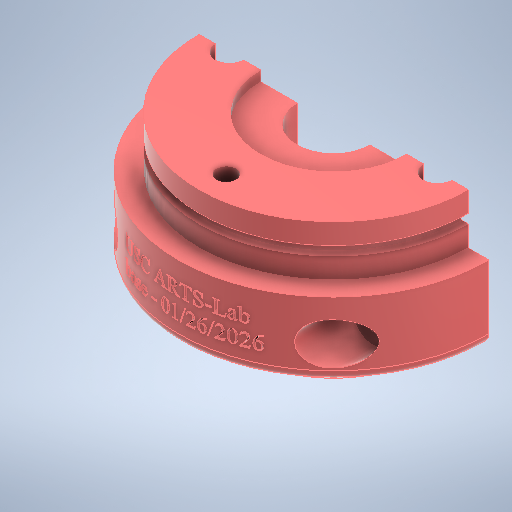
# Autodesk Inventor part: base_v0.7.0
Saved by Autodesk Inventor 2025 (Build 290162000, 162)
## iProperties
Created: 2026-01-12
Part Number: base_v0.7.0
Material: ABS Plastic
Document SubType Name: Modeling
Designer: SLM30
Density: 1.06 g/cm^3
Appearance: Smooth - Red
Author: SLM30
Autodesk Inventor part; units mm, degrees
ref_plane "YZ Plane" through (0, 0, 0) normal (1, 0, 0) x (0, 1, 0)
ref_plane "XZ Plane" through (0, 0, 0) normal (0, 1, 0) x (-1, 0, 0)
sketch "Sketch1" plane through (0, 0, 0) normal (0, 0, 1) x (1, 0, 0)
  line L0 (0, 0) -> (-14, 0)
  line L1 (-14, 0) -> (-14, 2)
  line L2 (-14, 2) -> (-25.825, 2)
  line L3 (-25.825, 2) -> (-25.825, -7.7)
  line L4 (-25.825, -7.7) -> (-29.825, -7.7)
  line L5 (0, 0) -> (0, -15)
  line L6 (0, -15) -> (-16, -15)
  line L7 (-16, -15) -> (-16, -26)
  line L8 (-16, -26) -> (0, -26)
  line L9 (0, -26) -> (0, -31)
  line L10 (0, -31) -> (-16, -31)
  line L11 (-29.825, -7.7) -> (-29.825, -21)
  line L12 (-29.825, -21) -> (-16, -31)
  arc A0 (-24.6268, -3.7009) -> (-24.6268, -2.0009) centre (-25.325, -2.8509) ccw
  line L13 (-25.825, -2.0009) -> (-24.6268, -2.0009)
  line L14 (-25.825, -3.7009) -> (-24.6268, -3.7009)
  line L15 (0, -37.6) -> (0, 8.6) projected
  dimension "d0" = 14
  dimension "d1" = 2
  dimension "d2" = 11.825
  dimension "d3" = 9.7
  dimension "d4" = 4
  dimension "d5" = 15
  dimension "d6" = 16
  dimension "d7" = 11
  dimension "d8" = 5
  dimension "d9" = 13.825
  dimension "d10" = 125.879
  dimension "d11" = 1.7
  dimension "d12" = 1.1
  dimension "d13" = 0.5
  dimension "d14" = 0.85
  dimension "d15" = 4.0009
  constraints: 30 end point, 7 perpendicular, 4 point on line, 3 horizontal, 2 point on circle, 2 vertical, 1 centre point, 1 parallel
  measures "d0" distance of L0.start L0.end
  measures "d1" distance of L0.end L1.end
  measures "d2" distance of L1.end L2.end
  measures "d3" distance of L2.end L3.end
  measures "d4" distance of L3.end L4.end
  measures "d5" distance of L0.start L5.end
  measures "d6" distance of L5.end L6.end
  measures "d7" distance of L6.end L7.end
  measures "d8" distance of L8.end L9.end
  measures "d9" horizontal distance of L11.end L10.end
  measures "d10" angle of L11 L12
  measures "d11" distance of L14.start L13.start
  measures "d12" radius of A0
  measures "d13" distance from line of L3 A0.centre
  measures "d14" distance from line of L14 A0.centre
  measures "d15" distance between parallel lines of L2 L13
revolve "Revolution1" add sketch "Sketch1" angle 180 about axis through (0, -10, 0) along (0, 1, 0) contours L5 L6 L7 L8 L9 L10 L12 L11 L4 L3 L14 A0 L13 L2 L1 L0
sketch "Sketch2" plane through (16, -31, 0) normal (0, 0, -1) x (-1, 0, 0)
  circle A0 centre (6, 10.5) radius 2.25
  line L0 (0, 5) -> (0, 16) projected
  line L1 (32, 16) -> (0, 16) projected
  point P0 (16, 31)
  dimension "d17" = 4.5
  dimension "d18" = 6
  dimension "d19" = 5.5
  constraints: 1 centre point
  measures "d17" diameter of A0
  measures "d18" distance from line of L0 A0.centre
  measures "d19" distance from line of L1 A0.centre
hole "Hole1" at (10, -20.5, 0) direction (0, 0, 1) diameter 4.5 depth 21.25
mirror "Mirror1" about plane through (0, 0, 0) normal (1, 0, 0) of "Hole1"
sketch "Sketch3" plane through (0, 0, 0) normal (0, 1, 0) x (1, 0, 0)
  circle A0 centre (0, 0) radius 7
  dimension "d27" = 14
  constraints: 1 centre point, 1 coincident
  measures "d27" diameter of A0
hole "Hole2" at (0, 0, 0) direction (0, -1, 0) diameter 14 depth 15
sketch "Sketch4" plane through (-16, -31, 0) normal (0, -1, 0) x (1, 0, 0)
  circle A0 centre (16, 0) radius 7
  point P0 (16, 0)
  dimension "d35" = 14
  constraints: 1 centre point, 1 coincident
  measures "d35" diameter of A0
hole "Hole3" at (0, -31, 0) direction (0, 1, 0) diameter 14 depth 10
ref_plane "Work Plane1" through (0, 0, 30) normal (0, 0, 1) x (1, 0, 0)
sketch "Sketch8" plane through (25.825, 2, 0) normal (0, 0, -1) x (-1, 0, 0)
  circle A0 centre (4.825, -17.5) radius 1.75
  line L0 (55.65, -23) -> (-4, -23) projected
  line L1 (9.825, -28) -> (9.825, -17) projected
  point P0 (25.825, -2)
  point P1 (-4, -23)
  dimension "d78" = 3.5
  dimension "d79" = 5.5
  dimension "d80" = 5
  constraints: 1 centre point, 1 other
  measures "d78" diameter of A0
  measures "d80" distance from line of L1 A0.centre
hole "Hole7" at (21, -15.5, 0) direction (0, 0, 1) diameter 3.5 end through all
mirror "Mirror2" about plane through (0, 0, 0) normal (1, 0, 0) of "Hole7"
sketch "Sketch9" plane through (0, 0, 30) normal (0, 0, 1) x (1, 0, 0)
  circle A0 centre (-21, -15.5) radius 1.75 projected
  circle A1 centre (-21, -15.5) radius 4
  point P0 (0, 0)
  dimension "d88" = 8
  constraints: 1 centre point, 1 coincident
  measures "d88" diameter of A1
hole "Hole8" at (-21, -15.5, 30) direction (0, 0, -1) diameter 8 depth 14
mirror "Mirror3" about plane through (0, 0, 0) normal (1, 0, 0) of "Hole8"
sketch "Sketch10" plane through (0, 0, 30) normal (0, 0, 1) x (1, 0, 0)
  circle A0 centre (-21, -15.5) radius 1.75 projected
  line L0 (-18.8265, -17.7354) -> (-21.8492, -18.5)
  line L1 (-21.8492, -18.5) -> (-24.0227, -16.2646)
  line L2 (-24.0227, -16.2646) -> (-23.1735, -13.2646)
  line L3 (-23.1735, -13.2646) -> (-20.1508, -12.5)
  line L4 (-20.1508, -12.5) -> (-17.9773, -14.7354)
  line L5 (-17.9773, -14.7354) -> (-18.8265, -17.7354)
  point P0 (0, 0)
  dimension "d135" = 3
  constraints: 12 end point, 1 coincident, 13 other
  measures "d135" vertical distance of L4.end L0.start
extrude "Extrusion1" cut sketch "Sketch10" against normal blind 16
fillet "Fillet1" radius 2 1 edges at (0, -21, 29.825)
sketch "Sketch16" plane through (-25.825, 2, 0) normal (0, 1, 0) x (1, 0, 0)
  circle A0 centre (25.825, -20.615) radius 1.9085
  arc A1 (0, 0) -> (51.65, 0) centre (25.825, 0) ccw projected
  point P0 (25.825, 0)
  point P1 (25.825, -25.825)
  dimension "d108" = 3.817
  dimension "d109" = 20.615
  dimension "d110" = 5.21
  constraints: 1 centre point, 1 point on circle
  measures "d108" diameter of A0
  measures "d109" distance of point (25.825, 0) A0.centre
  measures "d110" distance of point (25.825, -25.825) A0.centre
hole "Hole9" at (0, 2, 20.615) direction (0, -1, 0) diameter 3.817 end through all
sketch "Sketch17" plane through (-16, -31, 0) normal (0, -1, 0) x (1, 0, 0)
  circle A0 centre (16, 20.615) radius 1.9085 projected
  circle A1 centre (16, 20.615) radius 3
  point P0 (16, 0)
  dimension "d118" = 6
  constraints: 1 centre point, 1 coincident
  measures "d118" diameter of A1
hole "Hole10" at (0, -31, 20.615) direction (0, 1, 0) diameter 6 depth 7
sketch "Sketch18" plane through (-25.825, 2, 0) normal (0, 1, 0) x (1, 0, 0)
  circle A0 centre (5.825, 0) radius 2.75
  point P0 (25.825, 0)
  dimension "d126" = 5.5
  dimension "d127" = 20
  constraints: 1 centre point
  measures "d126" diameter of A0
  measures "d127" distance of point (25.825, 0) A0.centre
hole "Hole11" at (-20, 2, 0) direction (0, -1, 0) diameter 5.5 depth 3.3
mirror "Mirror5" about plane through (0, 0, 0) normal (1, 0, 0) of "Hole11"
move faces "Move1" translate (0, 0, -2.5) faces at (20.5413, -18.6943, 16) (17.0002, -15.4615, 18.8349)
ref_plane "Work Plane3" through (0, -14.35, 29.825) normal (0, 0, 1) x (1, 0, 0)
sketch "Sketch19" plane through (0, -14.35, 29.825) normal (0, 0, 1) x (1, 0, 0)
  line L0 (-29.825, 6.65) -> (-29.825, -5.6283) projected
  line L1 (-11.7404, 3.0074) -> (-11.7404, 3.0759)
  line L2 (-11.7404, 3.0759) -> (-10.846, 3.0759)
  line L3 (-10.846, 3.0759) -> (-10.846, 3.0074)
  line L4 (-10.846, 3.0074) -> (-10.9415, 3.0074)
  spline S0 degree 2 poles (-10.9415, 3.0074) (-11.0909, 3.0074) (-11.1697, 2.8808) knots 0 0 0 1 1 1
  spline S1 degree 2 poles (-11.1697, 2.8808) (-11.2092, 2.8227) (-11.2092, 2.611) knots 0 0 0 1 1 1
  line L5 (-11.2092, 2.611) -> (-11.2092, 1.5818)
  spline S2 degree 2 poles (-11.2092, 1.5818) (-11.2092, 1.1999) (-11.3606, 0.7787) (-11.8047, 0.4778) (-12.1866, 0.4778) knots 0 0 0 1 2 3 3 3
  spline S3 degree 2 poles (-12.1866, 0.4778) (-12.6016, 0.4778) (-13.0332, 0.7662) (-13.1225, 1.009) knots 0 0 0 1 2 2 2
  spline S4 degree 2 poles (-13.1225, 1.009) (-13.1826, 1.175) (-13.1826, 1.6336) knots 0 0 0 1 1 1
  line L6 (-13.1826, 1.6336) -> (-13.1826, 2.6256)
  spline S5 degree 2 poles (-13.1826, 2.6256) (-13.1826, 2.8601) (-13.3113, 3.0074) (-13.4566, 3.0074) knots 0 0 0 1 2 2 2
  line L7 (-13.4566, 3.0074) -> (-13.552, 3.0074)
  line L8 (-13.552, 3.0074) -> (-13.552, 3.0759)
  line L9 (-13.552, 3.0759) -> (-12.4543, 3.0759)
  line L10 (-12.4543, 3.0759) -> (-12.4543, 3.0074)
  line L11 (-12.4543, 3.0074) -> (-12.5518, 3.0074)
  spline S6 degree 2 poles (-12.5518, 3.0074) (-12.7095, 3.0074) (-12.7759, 2.9078) knots 0 0 0 1 1 1
  spline S7 degree 2 poles (-12.7759, 2.9078) (-12.8236, 2.8393) (-12.8236, 2.6256) knots 0 0 0 1 1 1
  line L12 (-12.8236, 2.6256) -> (-12.8236, 1.5195)
  spline S8 degree 2 poles (-12.8236, 1.5195) (-12.8236, 1.3722) (-12.7697, 0.9903) (-12.6265, 0.7787) (-12.3588, 0.6396) (-12.1637, 0.6396) knots 0 0 0 1 2 3 4 4 4
  spline S9 degree 2 poles (-12.1637, 0.6396) (-11.9147, 0.6396) (-11.5225, 0.8575) (-11.3772, 1.1958) (-11.3772, 1.5984) knots 0 0 0 1 2 3 3 3
  line L13 (-11.3772, 1.5984) -> (-11.3772, 2.6256)
  spline S10 degree 2 poles (-11.3772, 2.6256) (-11.3772, 2.8642) (-11.4291, 2.9244) knots 0 0 0 1 1 1
  spline S11 degree 2 poles (-11.4291, 2.9244) (-11.5018, 3.0074) (-11.6449, 3.0074) knots 0 0 0 1 1 1
  line L14 (-11.6449, 3.0074) -> (-11.7404, 3.0074)
  line L15 (-9.0385, 3.134) -> (-9.0385, 2.2562)
  line L16 (-9.0385, 2.2562) -> (-9.107, 2.2562)
  spline S12 degree 2 poles (-9.107, 2.2562) (-9.1402, 2.5094) (-9.3166, 2.8082) (-9.6383, 2.9846) (-9.8126, 2.9846) knots 0 0 0 1 2 3 3 3
  spline S13 degree 2 poles (-9.8126, 2.9846) (-10.0076, 2.9846) (-10.2629, 2.7459) (-10.2629, 2.5944) knots 0 0 0 1 2 2 2
  spline S14 degree 2 poles (-10.2629, 2.5944) (-10.2629, 2.4782) (-10.1819, 2.3828) knots 0 0 0 1 1 1
  spline S15 degree 2 poles (-10.1819, 2.3828) (-10.0657, 2.2417) (-9.6279, 2.0072) knots 0 0 0 1 1 1
  spline S16 degree 2 poles (-9.6279, 2.0072) (-9.273, 1.8163) (-9.0116, 1.6129) (-8.8704, 1.3348) (-8.8704, 1.1833) knots 0 0 0 1 2 3 3 3
  spline S17 degree 2 poles (-8.8704, 1.1833) (-8.8704, 0.8949) (-9.3187, 0.4778) (-9.6715, 0.4778) knots 0 0 0 1 2 2 2
  spline S18 degree 2 poles (-9.6715, 0.4778) (-9.7814, 0.4778) (-9.879, 0.4944) knots 0 0 0 1 1 1
  spline S19 degree 2 poles (-9.879, 0.4944) (-9.9371, 0.5048) (-10.3023, 0.623) (-10.3521, 0.623) knots 0 0 0 1 2 2 2
  spline S20 degree 2 poles (-10.3521, 0.623) (-10.3978, 0.623) (-10.4538, 0.567) (-10.4662, 0.4778) knots 0 0 0 1 2 2 2
  line L17 (-10.4662, 0.4778) -> (-10.5347, 0.4778)
  line L18 (-10.5347, 0.4778) -> (-10.5347, 1.3493)
  line L19 (-10.5347, 1.3493) -> (-10.4662, 1.3493)
  spline S21 degree 2 poles (-10.4662, 1.3493) (-10.4185, 1.0754) (-10.2525, 0.8036) (-9.9122, 0.623) (-9.7109, 0.623) knots 0 0 0 1 2 3 3 3
  spline S22 degree 2 poles (-9.7109, 0.623) (-9.4764, 0.623) (-9.2045, 0.87) (-9.2045, 1.0401) knots 0 0 0 1 2 2 2
  spline S23 degree 2 poles (-9.2045, 1.0401) (-9.2045, 1.1335) (-9.3083, 1.3244) (-9.4162, 1.4075) knots 0 0 0 1 2 2 2
  spline S24 degree 2 poles (-9.4162, 1.4075) (-9.4888, 1.4635) (-10.1425, 1.8287) (-10.4185, 2.0466) (-10.5617, 2.3081) (-10.5617, 2.4658) knots 0 0 0 1 2 3 4 4 4
  spline S25 degree 2 poles (-10.5617, 2.4658) (-10.5617, 2.7397) (-10.1404, 3.134) (-9.8146, 3.134) knots 0 0 0 1 2 2 2
  spline S26 degree 2 poles (-9.8146, 3.134) (-9.6134, 3.134) (-9.3851, 3.0344) knots 0 0 0 1 1 1
  spline S27 degree 2 poles (-9.3851, 3.0344) (-9.2793, 2.9887) (-9.2357, 2.9887) knots 0 0 0 1 1 1
  spline S28 degree 2 poles (-9.2357, 2.9887) (-9.1879, 2.9887) (-9.1257, 3.0468) (-9.107, 3.134) knots 0 0 0 1 2 2 2
  line L20 (-9.107, 3.134) -> (-9.0385, 3.134)
  line L21 (-6.3595, 3.134) -> (-6.3014, 2.2707)
  line L22 (-6.3014, 2.2707) -> (-6.3595, 2.2707)
  spline S29 degree 2 poles (-6.3595, 2.2707) (-6.4757, 2.6588) (-6.9053, 3.0012) (-7.2062, 3.0012) knots 0 0 0 1 2 2 2
  spline S30 degree 2 poles (-7.2062, 3.0012) (-7.4573, 3.0012) (-7.864, 2.7439) (-8.0985, 2.1815) (-8.0985, 1.7623) knots 0 0 0 1 2 3 3 3
  spline S31 degree 2 poles (-8.0985, 1.7623) (-8.0985, 1.4178) (-7.8785, 0.9115) (-7.4344, 0.6417) (-7.1522, 0.6417) knots 0 0 0 1 2 3 3 3
  spline S32 degree 2 poles (-7.1522, 0.6417) (-6.9053, 0.6417) (-6.5276, 0.8534) (-6.3014, 1.1688) knots 0 0 0 1 2 2 2
  line L23 (-6.3014, 1.1688) -> (-6.2433, 1.1315)
  spline S33 degree 2 poles (-6.2433, 1.1315) (-6.4342, 0.7932) (-6.9426, 0.4778) (-7.2933, 0.4778) knots 0 0 0 1 2 2 2
  spline S34 degree 2 poles (-7.2933, 0.4778) (-7.9242, 0.4778) (-8.2707, 0.9468) knots 0 0 0 1 1 1
  spline S35 degree 2 poles (-8.2707, 0.9468) (-8.528, 1.2954) (-8.528, 1.7665) knots 0 0 0 1 1 1
  spline S36 degree 2 poles (-8.528, 1.7665) (-8.528, 2.1462) (-8.1877, 2.7833) (-7.5901, 3.134) (-7.2373, 3.134) knots 0 0 0 1 2 3 3 3
  spline S37 degree 2 poles (-7.2373, 3.134) (-6.9634, 3.134) (-6.6957, 2.9991) knots 0 0 0 1 1 1
  spline S38 degree 2 poles (-6.6957, 2.9991) (-6.6168, 2.9576) (-6.5836, 2.9576) knots 0 0 0 1 1 1
  spline S39 degree 2 poles (-6.5836, 2.9576) (-6.5317, 2.9576) (-6.4944, 2.9929) knots 0 0 0 1 1 1
  spline S40 degree 2 poles (-6.4944, 2.9929) (-6.4467, 3.0448) (-6.4259, 3.134) knots 0 0 0 1 1 1
  line L24 (-6.4259, 3.134) -> (-6.3595, 3.134)
  line L25 (-3.392, 1.3846) -> (-4.3798, 1.3846)
  line L26 (-4.3798, 1.3846) -> (-4.552, 0.9862)
  spline S41 degree 2 poles (-4.552, 0.9862) (-4.6164, 0.8368) (-4.6164, 0.7641) knots 0 0 0 1 1 1
  spline S42 degree 2 poles (-4.6164, 0.7641) (-4.6164, 0.706) (-4.5043, 0.6168) (-4.3217, 0.6044) knots 0 0 0 1 2 2 2
  line L27 (-4.3217, 0.6044) -> (-4.3217, 0.5359)
  line L28 (-4.3217, 0.5359) -> (-5.1227, 0.5359)
  line L29 (-5.1227, 0.5359) -> (-5.1227, 0.6044)
  spline S43 degree 2 poles (-5.1227, 0.6044) (-4.9629, 0.6334) (-4.9173, 0.677) knots 0 0 0 1 1 1
  spline S44 degree 2 poles (-4.9173, 0.677) (-4.8218, 0.7683) (-4.7056, 1.0443) knots 0 0 0 1 1 1
  line L30 (-4.7056, 1.0443) -> (-3.8091, 3.134)
  line L31 (-3.8091, 3.134) -> (-3.7427, 3.134)
  line L32 (-3.7427, 3.134) -> (-2.8587, 1.0215)
  spline S45 degree 2 poles (-2.8587, 1.0215) (-2.7529, 0.7662) (-2.5786, 0.6147) (-2.4229, 0.6044) knots 0 0 0 1 2 2 2
  line L33 (-2.4229, 0.6044) -> (-2.4229, 0.5359)
  line L34 (-2.4229, 0.5359) -> (-3.4252, 0.5359)
  line L35 (-3.4252, 0.5359) -> (-3.4252, 0.6044)
  spline S46 degree 2 poles (-3.4252, 0.6044) (-3.2737, 0.6127) (-3.1658, 0.6977) (-3.1658, 0.76) knots 0 0 0 1 2 2 2
  spline S47 degree 2 poles (-3.1658, 0.76) (-3.1658, 0.843) (-3.2405, 1.0215) knots 0 0 0 1 1 1
  line L36 (-3.2405, 1.0215) -> (-3.392, 1.3846)
  line L37 (-3.4501, 1.5237) -> (-3.8776, 2.5509)
  line L38 (-3.8776, 2.5509) -> (-4.3217, 1.5237)
  line L39 (-4.3217, 1.5237) -> (-3.4501, 1.5237)
  line L40 (0.2125, 0.5359) -> (-0.466, 0.5359)
  line L41 (-0.466, 0.5359) -> (-1.3272, 1.7229)
  spline S48 degree 2 poles (-1.3272, 1.7229) (-1.4227, 1.7187) (-1.4808, 1.7187) knots 0 0 0 1 1 1
  spline S49 degree 2 poles (-1.4808, 1.7187) (-1.5057, 1.7187) (-1.5617, 1.7208) (-1.5908, 1.7229) knots 0 0 0 1 2 2 2
  line L42 (-1.5908, 1.7229) -> (-1.5908, 0.9862)
  spline S50 degree 2 poles (-1.5908, 0.9862) (-1.5908, 0.7455) (-1.5389, 0.6874) knots 0 0 0 1 1 1
  spline S51 degree 2 poles (-1.5389, 0.6874) (-1.4683, 0.6044) (-1.3272, 0.6044) knots 0 0 0 1 1 1
  line L43 (-1.3272, 0.6044) -> (-1.2276, 0.6044)
  line L44 (-1.2276, 0.6044) -> (-1.2276, 0.5359)
  line L45 (-1.2276, 0.5359) -> (-2.3129, 0.5359)
  line L46 (-2.3129, 0.5359) -> (-2.3129, 0.6044)
  line L47 (-2.3129, 0.6044) -> (-2.2175, 0.6044)
  spline S52 degree 2 poles (-2.2175, 0.6044) (-2.0577, 0.6044) (-1.9892, 0.7102) knots 0 0 0 1 1 1
  spline S53 degree 2 poles (-1.9892, 0.7102) (-1.9498, 0.7683) (-1.9498, 0.9862) knots 0 0 0 1 1 1
  line L48 (-1.9498, 0.9862) -> (-1.9498, 2.6256)
  spline S54 degree 2 poles (-1.9498, 2.6256) (-1.9498, 2.8663) (-2.0017, 2.9244) knots 0 0 0 1 1 1
  spline S55 degree 2 poles (-2.0017, 2.9244) (-2.0743, 3.0074) (-2.2175, 3.0074) knots 0 0 0 1 1 1
  line L49 (-2.2175, 3.0074) -> (-2.3129, 3.0074)
  line L50 (-2.3129, 3.0074) -> (-2.3129, 3.0759)
  line L51 (-2.3129, 3.0759) -> (-1.3895, 3.0759)
  spline S56 degree 2 poles (-1.3895, 3.0759) (-0.9848, 3.0759) (-0.6009, 2.9576) (-0.3332, 2.6422) (-0.3332, 2.4222) knots 0 0 0 1 2 3 3 3
  spline S57 degree 2 poles (-0.3332, 2.4222) (-0.3332, 2.1877) (-0.6383, 1.8432) (-0.9599, 1.7727) knots 0 0 0 1 2 2 2
  line L52 (-0.9599, 1.7727) -> (-0.4328, 1.0443)
  spline S58 degree 2 poles (-0.4328, 1.0443) (-0.2523, 0.7932) (0.005, 0.6272) (0.2125, 0.6044) knots 0 0 0 1 2 2 2
  line L53 (0.2125, 0.6044) -> (0.2125, 0.5359)
  spline S59 degree 2 poles (-1.5908, 1.8412) (-1.5555, 1.8412) (-1.5036, 1.8391) (-1.487, 1.8391) knots 0 0 0 1 2 2 2
  spline S60 degree 2 poles (-1.487, 1.8391) (-1.128, 1.8391) (-0.7628, 2.1545) (-0.7628, 2.3973) knots 0 0 0 1 2 2 2
  spline S61 degree 2 poles (-0.7628, 2.3973) (-0.7628, 2.6359) (-1.0575, 2.9327) (-1.3003, 2.9327) knots 0 0 0 1 2 2 2
  spline S62 degree 2 poles (-1.3003, 2.9327) (-1.4082, 2.9327) (-1.5908, 2.8974) knots 0 0 0 1 1 1
  line L54 (-1.5908, 2.8974) -> (-1.5908, 1.8412)
  line L55 (2.3956, 3.0759) -> (2.4226, 2.4803)
  line L56 (2.4226, 2.4803) -> (2.352, 2.4803)
  spline S63 degree 2 poles (2.352, 2.4803) (2.3313, 2.6359) (2.296, 2.7044) knots 0 0 0 1 1 1
  spline S64 degree 2 poles (2.296, 2.7044) (2.2379, 2.8123) (2.0449, 2.9161) (1.8872, 2.9161) knots 0 0 0 1 2 2 2
  line L57 (1.8872, 2.9161) -> (1.5303, 2.9161)
  line L58 (1.5303, 2.9161) -> (1.5303, 0.9758)
  spline S65 degree 2 poles (1.5303, 0.9758) (1.5303, 0.7413) (1.5801, 0.6832) knots 0 0 0 1 1 1
  spline S66 degree 2 poles (1.5801, 0.6832) (1.6527, 0.6044) (1.8, 0.6044) knots 0 0 0 1 1 1
  line L59 (1.8, 0.6044) -> (1.8872, 0.6044)
  line L60 (1.8872, 0.6044) -> (1.8872, 0.5359)
  line L61 (1.8872, 0.5359) -> (0.8123, 0.5359)
  line L62 (0.8123, 0.5359) -> (0.8123, 0.6044)
  line L63 (0.8123, 0.6044) -> (0.9015, 0.6044)
  spline S67 degree 2 poles (0.9015, 0.6044) (1.0634, 0.6044) (1.1298, 0.7019) knots 0 0 0 1 1 1
  spline S68 degree 2 poles (1.1298, 0.7019) (1.1713, 0.7621) (1.1713, 0.9758) knots 0 0 0 1 1 1
  line L64 (1.1713, 0.9758) -> (1.1713, 2.9161)
  line L65 (1.1713, 2.9161) -> (0.8662, 2.9161)
  spline S69 degree 2 poles (0.8662, 2.9161) (0.6878, 2.9161) (0.6131, 2.8891) knots 0 0 0 1 1 1
  spline S70 degree 2 poles (0.6131, 2.8891) (0.5155, 2.8538) (0.3786, 2.6525) (0.364, 2.4803) knots 0 0 0 1 2 2 2
  line L66 (0.364, 2.4803) -> (0.2935, 2.4803)
  line L67 (0.2935, 2.4803) -> (0.3225, 3.0759)
  line L68 (0.3225, 3.0759) -> (2.3956, 3.0759)
  line L69 (4.284, 3.134) -> (4.284, 2.2562)
  line L70 (4.284, 2.2562) -> (4.2155, 2.2562)
  spline S71 degree 2 poles (4.2155, 2.2562) (4.1823, 2.5094) (4.0059, 2.8082) (3.6843, 2.9846) (3.51, 2.9846) knots 0 0 0 1 2 3 3 3
  spline S72 degree 2 poles (3.51, 2.9846) (3.3149, 2.9846) (3.0597, 2.7459) (3.0597, 2.5944) knots 0 0 0 1 2 2 2
  spline S73 degree 2 poles (3.0597, 2.5944) (3.0597, 2.4782) (3.1406, 2.3828) knots 0 0 0 1 1 1
  spline S74 degree 2 poles (3.1406, 2.3828) (3.2568, 2.2417) (3.6947, 2.0072) knots 0 0 0 1 1 1
  spline S75 degree 2 poles (3.6947, 2.0072) (4.0495, 1.8163) (4.311, 1.6129) (4.4521, 1.3348) (4.4521, 1.1833) knots 0 0 0 1 2 3 3 3
  spline S76 degree 2 poles (4.4521, 1.1833) (4.4521, 0.8949) (4.0039, 0.4778) (3.6511, 0.4778) knots 0 0 0 1 2 2 2
  spline S77 degree 2 poles (3.6511, 0.4778) (3.5411, 0.4778) (3.4436, 0.4944) knots 0 0 0 1 1 1
  spline S78 degree 2 poles (3.4436, 0.4944) (3.3855, 0.5048) (3.0202, 0.623) (2.9704, 0.623) knots 0 0 0 1 2 2 2
  spline S79 degree 2 poles (2.9704, 0.623) (2.9248, 0.623) (2.8688, 0.567) (2.8563, 0.4778) knots 0 0 0 1 2 2 2
  line L71 (2.8563, 0.4778) -> (2.7878, 0.4778)
  line L72 (2.7878, 0.4778) -> (2.7878, 1.3493)
  line L73 (2.7878, 1.3493) -> (2.8563, 1.3493)
  spline S80 degree 2 poles (2.8563, 1.3493) (2.904, 1.0754) (3.07, 0.8036) (3.4104, 0.623) (3.6117, 0.623) knots 0 0 0 1 2 3 3 3
  spline S81 degree 2 poles (3.6117, 0.623) (3.8462, 0.623) (4.118, 0.87) (4.118, 1.0401) knots 0 0 0 1 2 2 2
  spline S82 degree 2 poles (4.118, 1.0401) (4.118, 1.1335) (4.0142, 1.3244) (3.9063, 1.4075) knots 0 0 0 1 2 2 2
  spline S83 degree 2 poles (3.9063, 1.4075) (3.8337, 1.4635) (3.18, 1.8287) (2.904, 2.0466) (2.7608, 2.3081) (2.7608, 2.4658) knots 0 0 0 1 2 3 4 4 4
  spline S84 degree 2 poles (2.7608, 2.4658) (2.7608, 2.7397) (3.1821, 3.134) (3.5079, 3.134) knots 0 0 0 1 2 2 2
  spline S85 degree 2 poles (3.5079, 3.134) (3.7092, 3.134) (3.9375, 3.0344) knots 0 0 0 1 1 1
  spline S86 degree 2 poles (3.9375, 3.0344) (4.0433, 2.9887) (4.0869, 2.9887) knots 0 0 0 1 1 1
  spline S87 degree 2 poles (4.0869, 2.9887) (4.1346, 2.9887) (4.1969, 3.0468) (4.2155, 3.134) knots 0 0 0 1 2 2 2
  line L74 (4.2155, 3.134) -> (4.284, 3.134)
  line L75 (4.809, 1.5382) -> (5.7802, 1.5382)
  line L76 (5.7802, 1.5382) -> (5.7802, 1.256)
  line L77 (5.7802, 1.256) -> (4.809, 1.256)
  line L78 (4.809, 1.256) -> (4.809, 1.5382)
  line L79 (8.1314, 1.2394) -> (8.1936, 1.2269)
  line L80 (8.1936, 1.2269) -> (7.9757, 0.5359)
  line L81 (7.9757, 0.5359) -> (6.0106, 0.5359)
  line L82 (6.0106, 0.5359) -> (6.0106, 0.6044)
  line L83 (6.0106, 0.6044) -> (6.106, 0.6044)
  spline S88 degree 2 poles (6.106, 0.6044) (6.2658, 0.6044) (6.3343, 0.7102) knots 0 0 0 1 1 1
  spline S89 degree 2 poles (6.3343, 0.7102) (6.3737, 0.7683) (6.3737, 0.9862) knots 0 0 0 1 1 1
  line L84 (6.3737, 0.9862) -> (6.3737, 2.6256)
  spline S90 degree 2 poles (6.3737, 2.6256) (6.3737, 2.8642) (6.3218, 2.9244) knots 0 0 0 1 1 1
  spline S91 degree 2 poles (6.3218, 2.9244) (6.2492, 3.0074) (6.106, 3.0074) knots 0 0 0 1 1 1
  line L85 (6.106, 3.0074) -> (6.0106, 3.0074)
  line L86 (6.0106, 3.0074) -> (6.0106, 3.0759)
  line L87 (6.0106, 3.0759) -> (7.1581, 3.0759)
  line L88 (7.1581, 3.0759) -> (7.1581, 3.0074)
  spline S92 degree 2 poles (7.1581, 3.0074) (6.9548, 3.0095) (6.7929, 2.9306) (6.7327, 2.8103) (6.7327, 2.5841) knots 0 0 0 1 2 3 3 3
  line L89 (6.7327, 2.5841) -> (6.7327, 0.9883)
  spline S93 degree 2 poles (6.7327, 0.9883) (6.7327, 0.8326) (6.7618, 0.7745) knots 0 0 0 1 1 1
  spline S94 degree 2 poles (6.7618, 0.7745) (6.7846, 0.7351) (6.878, 0.6977) (7.1249, 0.6977) knots 0 0 0 1 2 2 2
  line L90 (7.1249, 0.6977) -> (7.3096, 0.6977)
  spline S95 degree 2 poles (7.3096, 0.6977) (7.6022, 0.6977) (7.8388, 0.7849) (8.0338, 1.0028) (8.1314, 1.2394) knots 0 0 0 1 2 3 3 3
  spline S96 degree 2 poles (9.3661, 0.7849) (9.1025, 0.5795) (9.0341, 0.5483) knots 0 0 0 1 1 1
  spline S97 degree 2 poles (9.0341, 0.5483) (8.9345, 0.5006) (8.8203, 0.5006) knots 0 0 0 1 1 1
  spline S98 degree 2 poles (8.8203, 0.5006) (8.6419, 0.5006) (8.4115, 0.7434) (8.4115, 0.9426) knots 0 0 0 1 2 2 2
  spline S99 degree 2 poles (8.4115, 0.9426) (8.4115, 1.0671) (8.4675, 1.1605) knots 0 0 0 1 1 1
  spline S100 degree 2 poles (8.4675, 1.1605) (8.5443, 1.2871) (8.9241, 1.5112) (9.3661, 1.6731) knots 0 0 0 1 2 2 2
  line L91 (9.3661, 1.6731) -> (9.3661, 1.7395)
  spline S101 degree 2 poles (9.3661, 1.7395) (9.3661, 1.9968) (9.2042, 2.1877) (9.0486, 2.1877) knots 0 0 0 1 2 2 2
  spline S102 degree 2 poles (9.0486, 2.1877) (8.9324, 2.1877) (8.8618, 2.1234) knots 0 0 0 1 1 1
  spline S103 degree 2 poles (8.8618, 2.1234) (8.7913, 2.0611) (8.7913, 1.9781) knots 0 0 0 1 1 1
  line L92 (8.7913, 1.9781) -> (8.7954, 1.8702)
  spline S104 degree 2 poles (8.7954, 1.8702) (8.7954, 1.7831) (8.7062, 1.6897) (8.6356, 1.6897) knots 0 0 0 1 2 2 2
  spline S105 degree 2 poles (8.6356, 1.6897) (8.5672, 1.6897) (8.4779, 1.7872) (8.4779, 1.8723) knots 0 0 0 1 2 2 2
  spline S106 degree 2 poles (8.4779, 1.8723) (8.4779, 2.0321) (8.8079, 2.3018) (9.1046, 2.3018) knots 0 0 0 1 2 2 2
  spline S107 degree 2 poles (9.1046, 2.3018) (9.3329, 2.3018) (9.4781, 2.2251) knots 0 0 0 1 1 1
  spline S108 degree 2 poles (9.4781, 2.2251) (9.5902, 2.167) (9.6421, 2.0445) knots 0 0 0 1 1 1
  spline S109 degree 2 poles (9.6421, 2.0445) (9.6753, 1.9636) (9.6753, 1.7146) knots 0 0 0 1 1 1
  line L93 (9.6753, 1.7146) -> (9.6753, 1.1315)
  spline S110 degree 2 poles (9.6753, 1.1315) (9.6753, 0.8866) (9.694, 0.7766) (9.7375, 0.7392) (9.7645, 0.7392) knots 0 0 0 1 2 3 3 3
  spline S111 degree 2 poles (9.7645, 0.7392) (9.7956, 0.7392) (9.8185, 0.7517) knots 0 0 0 1 1 1
  spline S112 degree 2 poles (9.8185, 0.7517) (9.8579, 0.7766) (9.97, 0.8887) knots 0 0 0 1 1 1
  line L94 (9.97, 0.8887) -> (9.97, 0.7849)
  spline S113 degree 2 poles (9.97, 0.7849) (9.7604, 0.5027) (9.5695, 0.5027) knots 0 0 0 1 1 1
  spline S114 degree 2 poles (9.5695, 0.5027) (9.4761, 0.5027) (9.3682, 0.6293) (9.3661, 0.7849) knots 0 0 0 1 2 2 2
  line L95 (9.3661, 0.9053) -> (9.3661, 1.5589)
  spline S115 degree 2 poles (9.3661, 1.5589) (9.0839, 1.4469) (9.0009, 1.3991) knots 0 0 0 1 1 1
  spline S116 degree 2 poles (9.0009, 1.3991) (8.8535, 1.3182) (8.7269, 1.1377) (8.7269, 1.0318) knots 0 0 0 1 2 2 2
  spline S117 degree 2 poles (8.7269, 1.0318) (8.7269, 0.897) (8.8867, 0.7185) (8.9926, 0.7185) knots 0 0 0 1 2 2 2
  spline S118 degree 2 poles (8.9926, 0.7185) (9.1337, 0.7185) (9.3661, 0.9053) knots 0 0 0 1 1 1
  spline S119 degree 2 poles (10.5697, 1.9532) (10.8187, 2.3018) (11.1051, 2.3018) knots 0 0 0 1 1 1
  spline S120 degree 2 poles (11.1051, 2.3018) (11.3686, 2.3018) (11.7608, 1.8515) (11.7608, 1.4593) knots 0 0 0 1 2 2 2
  spline S121 degree 2 poles (11.7608, 1.4593) (11.7608, 1.0028) (11.4579, 0.7226) knots 0 0 0 1 1 1
  spline S122 degree 2 poles (11.4579, 0.7226) (11.1985, 0.484) (10.8768, 0.484) knots 0 0 0 1 1 1
  spline S123 degree 2 poles (10.8768, 0.484) (10.7274, 0.484) (10.4203, 0.5919) (10.2584, 0.7019) knots 0 0 0 1 2 2 2
  line L96 (10.2584, 0.7019) -> (10.2584, 2.4782)
  spline S124 degree 2 poles (10.2584, 2.4782) (10.2584, 2.7688) (10.2294, 2.9036) (10.1713, 2.9514) (10.1256, 2.9514) knots 0 0 0 1 2 3 3 3
  spline S125 degree 2 poles (10.1256, 2.9514) (10.0737, 2.9514) (9.9949, 2.9223) knots 0 0 0 1 1 1
  line L97 (9.9949, 2.9223) -> (9.9679, 2.9908)
  line L98 (9.9679, 2.9908) -> (10.4846, 3.2004)
  line L99 (10.4846, 3.2004) -> (10.5697, 3.2004)
  line L100 (10.5697, 3.2004) -> (10.5697, 1.9532)
  line L101 (10.5697, 1.8349) -> (10.5697, 0.8098)
  spline S126 degree 2 poles (10.5697, 0.8098) (10.6651, 0.7164) (10.8685, 0.621) (10.9743, 0.621) knots 0 0 0 1 2 2 2
  spline S127 degree 2 poles (10.9743, 0.621) (11.1445, 0.621) (11.4371, 0.9945) (11.4371, 1.3514) knots 0 0 0 1 2 2 2
  spline S128 degree 2 poles (11.4371, 1.3514) (11.4371, 1.6814) (11.1445, 2.0341) (10.9577, 2.0341) knots 0 0 0 1 2 2 2
  spline S129 degree 2 poles (10.9577, 2.0341) (10.8581, 2.0341) (10.7606, 1.9843) knots 0 0 0 1 1 1
  spline S130 degree 2 poles (10.7606, 1.9843) (10.6859, 1.947) (10.5697, 1.8349) knots 0 0 0 1 1 1
  spline S131 degree 2 poles (-12.9813, -2.0642) (-12.7323, -1.7155) (-12.446, -1.7155) knots 0 0 0 1 1 1
  spline S132 degree 2 poles (-12.446, -1.7155) (-12.1824, -1.7155) (-11.7902, -2.1658) (-11.7902, -2.558) knots 0 0 0 1 2 2 2
  spline S133 degree 2 poles (-11.7902, -2.558) (-11.7902, -3.0146) (-12.0932, -3.2947) knots 0 0 0 1 1 1
  spline S134 degree 2 poles (-12.0932, -3.2947) (-12.3526, -3.5334) (-12.6742, -3.5334) knots 0 0 0 1 1 1
  spline S135 degree 2 poles (-12.6742, -3.5334) (-12.8236, -3.5334) (-13.1308, -3.4255) (-13.2926, -3.3155) knots 0 0 0 1 2 2 2
  line L102 (-13.2926, -3.3155) -> (-13.2926, -1.5391)
  spline S136 degree 2 poles (-13.2926, -1.5391) (-13.2926, -1.2486) (-13.3217, -1.1137) (-13.3798, -1.066) (-13.4254, -1.066) knots 0 0 0 1 2 3 3 3
  spline S137 degree 2 poles (-13.4254, -1.066) (-13.4773, -1.066) (-13.5562, -1.0951) knots 0 0 0 1 1 1
  line L103 (-13.5562, -1.0951) -> (-13.5831, -1.0266)
  line L104 (-13.5831, -1.0266) -> (-13.0664, -0.817)
  line L105 (-13.0664, -0.817) -> (-12.9813, -0.817)
  line L106 (-12.9813, -0.817) -> (-12.9813, -2.0642)
  line L107 (-12.9813, -2.1824) -> (-12.9813, -3.2076)
  spline S138 degree 2 poles (-12.9813, -3.2076) (-12.8859, -3.301) (-12.6825, -3.3964) (-12.5767, -3.3964) knots 0 0 0 1 2 2 2
  spline S139 degree 2 poles (-12.5767, -3.3964) (-12.4065, -3.3964) (-12.1139, -3.0229) (-12.1139, -2.666) knots 0 0 0 1 2 2 2
  spline S140 degree 2 poles (-12.1139, -2.666) (-12.1139, -2.336) (-12.4065, -1.9832) (-12.5933, -1.9832) knots 0 0 0 1 2 2 2
  spline S141 degree 2 poles (-12.5933, -1.9832) (-12.6929, -1.9832) (-12.7904, -2.033) knots 0 0 0 1 1 1
  spline S142 degree 2 poles (-12.7904, -2.033) (-12.8651, -2.0704) (-12.9813, -2.1824) knots 0 0 0 1 1 1
  spline S143 degree 2 poles (-10.5617, -3.2325) (-10.8253, -3.4379) (-10.8937, -3.469) knots 0 0 0 1 1 1
  spline S144 degree 2 poles (-10.8937, -3.469) (-10.9933, -3.5168) (-11.1075, -3.5168) knots 0 0 0 1 1 1
  spline S145 degree 2 poles (-11.1075, -3.5168) (-11.2859, -3.5168) (-11.5163, -3.274) (-11.5163, -3.0748) knots 0 0 0 1 2 2 2
  spline S146 degree 2 poles (-11.5163, -3.0748) (-11.5163, -2.9502) (-11.4603, -2.8569) knots 0 0 0 1 1 1
  spline S147 degree 2 poles (-11.4603, -2.8569) (-11.3835, -2.7303) (-11.0037, -2.5062) (-10.5617, -2.3443) knots 0 0 0 1 2 2 2
  line L108 (-10.5617, -2.3443) -> (-10.5617, -2.2779)
  spline S148 degree 2 poles (-10.5617, -2.2779) (-10.5617, -2.0206) (-10.7236, -1.8297) (-10.8792, -1.8297) knots 0 0 0 1 2 2 2
  spline S149 degree 2 poles (-10.8792, -1.8297) (-10.9954, -1.8297) (-11.066, -1.894) knots 0 0 0 1 1 1
  spline S150 degree 2 poles (-11.066, -1.894) (-11.1365, -1.9562) (-11.1365, -2.0393) knots 0 0 0 1 1 1
  line L109 (-11.1365, -2.0393) -> (-11.1324, -2.1472)
  spline S151 degree 2 poles (-11.1324, -2.1472) (-11.1324, -2.2343) (-11.2216, -2.3277) (-11.2922, -2.3277) knots 0 0 0 1 2 2 2
  spline S152 degree 2 poles (-11.2922, -2.3277) (-11.3606, -2.3277) (-11.4499, -2.2302) (-11.4499, -2.1451) knots 0 0 0 1 2 2 2
  spline S153 degree 2 poles (-11.4499, -2.1451) (-11.4499, -1.9853) (-11.1199, -1.7155) (-10.8232, -1.7155) knots 0 0 0 1 2 2 2
  spline S154 degree 2 poles (-10.8232, -1.7155) (-10.5949, -1.7155) (-10.4496, -1.7923) knots 0 0 0 1 1 1
  spline S155 degree 2 poles (-10.4496, -1.7923) (-10.3376, -1.8504) (-10.2857, -1.9728) knots 0 0 0 1 1 1
  spline S156 degree 2 poles (-10.2857, -1.9728) (-10.2525, -2.0538) (-10.2525, -2.3028) knots 0 0 0 1 1 1
  line L110 (-10.2525, -2.3028) -> (-10.2525, -2.8859)
  spline S157 degree 2 poles (-10.2525, -2.8859) (-10.2525, -3.1308) (-10.2338, -3.2408) (-10.1903, -3.2781) (-10.1633, -3.2781) knots 0 0 0 1 2 3 3 3
  spline S158 degree 2 poles (-10.1633, -3.2781) (-10.1321, -3.2781) (-10.1093, -3.2657) knots 0 0 0 1 1 1
  spline S159 degree 2 poles (-10.1093, -3.2657) (-10.0699, -3.2408) (-9.9578, -3.1287) knots 0 0 0 1 1 1
  line L111 (-9.9578, -3.1287) -> (-9.9578, -3.2325)
  spline S160 degree 2 poles (-9.9578, -3.2325) (-10.1674, -3.5147) (-10.3583, -3.5147) knots 0 0 0 1 1 1
  spline S161 degree 2 poles (-10.3583, -3.5147) (-10.4517, -3.5147) (-10.5596, -3.3881) (-10.5617, -3.2325) knots 0 0 0 1 2 2 2
  line L112 (-10.5617, -3.1121) -> (-10.5617, -2.4584)
  spline S162 degree 2 poles (-10.5617, -2.4584) (-10.8439, -2.5705) (-10.9269, -2.6182) knots 0 0 0 1 1 1
  spline S163 degree 2 poles (-10.9269, -2.6182) (-11.0743, -2.6992) (-11.2009, -2.8797) (-11.2009, -2.9855) knots 0 0 0 1 2 2 2
  spline S164 degree 2 poles (-11.2009, -2.9855) (-11.2009, -3.1204) (-11.0411, -3.2989) (-10.9352, -3.2989) knots 0 0 0 1 2 2 2
  spline S165 degree 2 poles (-10.9352, -3.2989) (-10.7941, -3.2989) (-10.5617, -3.1121) knots 0 0 0 1 1 1
  line L113 (-8.721, -1.7155) -> (-8.721, -2.3007)
  line L114 (-8.721, -2.3007) -> (-8.7833, -2.3007)
  spline S166 degree 2 poles (-8.7833, -2.3007) (-8.8538, -2.0247) (-9.0759, -1.8255) (-9.2481, -1.8255) knots 0 0 0 1 2 2 2
  spline S167 degree 2 poles (-9.2481, -1.8255) (-9.3789, -1.8255) (-9.5407, -1.9645) (-9.5407, -2.0476) knots 0 0 0 1 2 2 2
  spline S168 degree 2 poles (-9.5407, -2.0476) (-9.5407, -2.1534) (-9.4805, -2.2281) knots 0 0 0 1 1 1
  spline S169 degree 2 poles (-9.4805, -2.2281) (-9.4245, -2.3049) (-9.2461, -2.392) knots 0 0 0 1 1 1
  line L115 (-9.2461, -2.392) -> (-8.9721, -2.5248)
  spline S170 degree 2 poles (-8.9721, -2.5248) (-8.5924, -2.7095) (-8.5924, -3.0125) knots 0 0 0 1 1 1
  spline S171 degree 2 poles (-8.5924, -3.0125) (-8.5924, -3.247) (-8.9452, -3.5334) (-9.1651, -3.5334) knots 0 0 0 1 2 2 2
  spline S172 degree 2 poles (-9.1651, -3.5334) (-9.3228, -3.5334) (-9.5241, -3.4773) knots 0 0 0 1 1 1
  spline S173 degree 2 poles (-9.5241, -3.4773) (-9.5864, -3.4587) (-9.6258, -3.4587) knots 0 0 0 1 1 1
  spline S174 degree 2 poles (-9.6258, -3.4587) (-9.6673, -3.4587) (-9.6922, -3.5064) knots 0 0 0 1 1 1
  line L116 (-9.6922, -3.5064) -> (-9.7545, -3.5064)
  line L117 (-9.7545, -3.5064) -> (-9.7545, -2.8942)
  line L118 (-9.7545, -2.8942) -> (-9.6922, -2.8942)
  spline S175 degree 2 poles (-9.6922, -2.8942) (-9.6403, -3.1578) (-9.3457, -3.4234) (-9.161, -3.4234) knots 0 0 0 1 2 2 2
  spline S176 degree 2 poles (-9.161, -3.4234) (-9.0323, -3.4234) (-8.8704, -3.2719) (-8.8704, -3.164) knots 0 0 0 1 2 2 2
  spline S177 degree 2 poles (-8.8704, -3.164) (-8.8704, -3.0353) (-9.051, -2.8589) (-9.5947, -2.5912) (-9.6798, -2.4813) knots 0 0 0 1 2 3 3 3
  spline S178 degree 2 poles (-9.6798, -2.4813) (-9.7628, -2.3754) (-9.7628, -2.2115) knots 0 0 0 1 1 1
  spline S179 degree 2 poles (-9.7628, -2.2115) (-9.7628, -1.9998) (-9.4722, -1.7155) (-9.2419, -1.7155) knots 0 0 0 1 2 2 2
  spline S180 degree 2 poles (-9.2419, -1.7155) (-9.1402, -1.7155) (-8.997, -1.7591) knots 0 0 0 1 1 1
  spline S181 degree 2 poles (-8.997, -1.7591) (-8.9016, -1.7861) (-8.8704, -1.7861) knots 0 0 0 1 1 1
  spline S182 degree 2 poles (-8.8704, -1.7861) (-8.8393, -1.7861) (-8.8061, -1.7591) (-8.7833, -1.7155) knots 0 0 0 1 2 2 2
  line L119 (-8.7833, -1.7155) -> (-8.721, -1.7155)
  spline S183 degree 2 poles (-8.0466, -2.4128) (-8.0487, -2.7946) (-7.8619, -3.0104) knots 0 0 0 1 1 1
  spline S184 degree 2 poles (-7.8619, -3.0104) (-7.6731, -3.2283) (-7.4199, -3.2283) knots 0 0 0 1 1 1
  spline S185 degree 2 poles (-7.4199, -3.2283) (-7.2518, -3.2283) (-7.0028, -3.0436) (-6.9177, -2.8174) knots 0 0 0 1 2 2 2
  line L120 (-6.9177, -2.8174) -> (-6.8596, -2.8548)
  spline S186 degree 2 poles (-6.8596, -2.8548) (-6.899, -3.1121) (-7.2767, -3.5334) (-7.5631, -3.5334) knots 0 0 0 1 2 2 2
  spline S187 degree 2 poles (-7.5631, -3.5334) (-7.8723, -3.5334) (-8.3122, -3.0519) (-8.3122, -2.6473) knots 0 0 0 1 2 2 2
  spline S188 degree 2 poles (-8.3122, -2.6473) (-8.3122, -2.2073) (-7.8598, -1.7155) (-7.5195, -1.7155) knots 0 0 0 1 2 2 2
  spline S189 degree 2 poles (-7.5195, -1.7155) (-7.2311, -1.7155) (-6.8596, -2.0953) (-6.8596, -2.4128) knots 0 0 0 1 2 2 2
  line L121 (-6.8596, -2.4128) -> (-8.0466, -2.4128)
  line L122 (-8.0466, -2.3049) -> (-7.2497, -2.3049)
  spline S190 degree 2 poles (-7.2497, -2.3049) (-7.2601, -2.1409) (-7.2892, -2.0725) knots 0 0 0 1 1 1
  spline S191 degree 2 poles (-7.2892, -2.0725) (-7.3369, -1.9687) (-7.5216, -1.8483) (-7.6233, -1.8483) knots 0 0 0 1 2 2 2
  spline S192 degree 2 poles (-7.6233, -1.8483) (-7.7789, -1.8483) (-8.0259, -2.0891) (-8.0466, -2.3049) knots 0 0 0 1 2 2 2
  line L123 (-5.6373, -2.4792) -> (-4.6662, -2.4792)
  line L124 (-4.6662, -2.4792) -> (-4.6662, -2.7614)
  line L125 (-4.6662, -2.7614) -> (-5.6373, -2.7614)
  line L126 (-5.6373, -2.7614) -> (-5.6373, -2.4792)
  spline S193 degree 2 poles (-3.4169, -2.226) (-3.4169, -1.7923) (-3.1554, -1.1656) (-2.9376, -1.012) knots 0 0 0 1 2 2 2
  spline S194 degree 2 poles (-2.9376, -1.012) (-2.7695, -0.8896) (-2.5889, -0.8896) knots 0 0 0 1 1 1
  spline S195 degree 2 poles (-2.5889, -0.8896) (-2.2963, -0.8896) (-2.0639, -1.1864) knots 0 0 0 1 1 1
  spline S196 degree 2 poles (-2.0639, -1.1864) (-1.7734, -1.5557) (-1.7734, -2.1866) knots 0 0 0 1 1 1
  spline S197 degree 2 poles (-1.7734, -2.1866) (-1.7734, -2.6286) (-2.0286, -3.247) (-2.4229, -3.5251) (-2.6076, -3.5251) knots 0 0 0 1 2 3 3 3
  spline S198 degree 2 poles (-2.6076, -3.5251) (-2.9708, -3.5251) (-3.2136, -3.0955) knots 0 0 0 1 1 1
  spline S199 degree 2 poles (-3.2136, -3.0955) (-3.4169, -2.7344) (-3.4169, -2.226) knots 0 0 0 1 1 1
  spline S200 degree 2 poles (-3.0496, -2.2737) (-3.0496, -2.7967) (-2.921, -3.1287) knots 0 0 0 1 1 1
  spline S201 degree 2 poles (-2.921, -3.1287) (-2.813, -3.4068) (-2.6014, -3.4068) knots 0 0 0 1 1 1
  spline S202 degree 2 poles (-2.6014, -3.4068) (-2.4997, -3.4068) (-2.2839, -3.2262) (-2.2278, -3.0125) knots 0 0 0 1 2 2 2
  spline S203 degree 2 poles (-2.2278, -3.0125) (-2.1407, -2.6909) (-2.1407, -2.1057) knots 0 0 0 1 1 1
  spline S204 degree 2 poles (-2.1407, -2.1057) (-2.1407, -1.6699) (-2.2299, -1.3814) knots 0 0 0 1 1 1
  spline S205 degree 2 poles (-2.2299, -1.3814) (-2.2984, -1.1656) (-2.4042, -1.0764) knots 0 0 0 1 1 1
  spline S206 degree 2 poles (-2.4042, -1.0764) (-2.481, -1.0141) (-2.591, -1.0141) knots 0 0 0 1 1 1
  spline S207 degree 2 poles (-2.591, -1.0141) (-2.7176, -1.0141) (-2.8172, -1.1283) knots 0 0 0 1 1 1
  spline S208 degree 2 poles (-2.8172, -1.1283) (-2.9521, -1.2839) (-3.0496, -1.95) (-3.0496, -2.2737) knots 0 0 0 1 2 2 2
  line L127 (-1.1882, -1.1905) -> (-0.5698, -0.8896)
  line L128 (-0.5698, -0.8896) -> (-0.5075, -0.8896)
  line L129 (-0.5075, -0.8896) -> (-0.5075, -3.0333)
  spline S209 degree 2 poles (-0.5075, -3.0333) (-0.5075, -3.247) (-0.4723, -3.3528) (-0.3602, -3.4089) (-0.188, -3.413) knots 0 0 0 1 2 3 3 3
  line L130 (-0.188, -3.413) -> (-0.188, -3.4815)
  line L131 (-0.188, -3.4815) -> (-1.1425, -3.4815)
  line L132 (-1.1425, -3.4815) -> (-1.1425, -3.413)
  spline S210 degree 2 poles (-1.1425, -3.413) (-0.962, -3.4089) (-0.8582, -3.3549) (-0.8167, -3.2636) (-0.8167, -3.0333) knots 0 0 0 1 2 3 3 3
  line L133 (-0.8167, -3.0333) -> (-0.8167, -1.6636)
  spline S211 degree 2 poles (-0.8167, -1.6636) (-0.8167, -1.3856) (-0.8354, -1.3067) knots 0 0 0 1 1 1
  spline S212 degree 2 poles (-0.8354, -1.3067) (-0.8479, -1.2465) (-0.9184, -1.1905) (-0.9661, -1.1905) knots 0 0 0 1 2 2 2
  spline S213 degree 2 poles (-0.9661, -1.1905) (-1.0367, -1.1905) (-1.1591, -1.2486) knots 0 0 0 1 1 1
  line L134 (-1.1591, -1.2486) -> (-1.1882, -1.1905)
  line L135 (1.356, -0.817) -> (0.4367, -3.5334)
  line L136 (0.4367, -3.5334) -> (0.2872, -3.5334)
  line L137 (0.2872, -3.5334) -> (1.2065, -0.817)
  line L138 (1.2065, -0.817) -> (1.356, -0.817)
  line L139 (3.1095, -2.9938) -> (2.931, -3.4815)
  line L140 (2.931, -3.4815) -> (1.4327, -3.4815)
  line L141 (1.4327, -3.4815) -> (1.4327, -3.413)
  spline S214 degree 2 poles (1.4327, -3.413) (2.0947, -2.8091) (2.6343, -2.0455) (2.6343, -1.728) knots 0 0 0 1 2 2 2
  spline S215 degree 2 poles (2.6343, -1.728) (2.6343, -1.4873) (2.3375, -1.176) (2.1321, -1.176) knots 0 0 0 1 2 2 2
  spline S216 degree 2 poles (2.1321, -1.176) (1.9432, -1.176) (1.6465, -1.396) (1.5739, -1.6076) knots 0 0 0 1 2 2 2
  line L142 (1.5739, -1.6076) -> (1.5054, -1.6076)
  spline S217 degree 2 poles (1.5054, -1.6076) (1.5531, -1.2611) (1.9391, -0.8896) (2.2296, -0.8896) knots 0 0 0 1 2 2 2
  spline S218 degree 2 poles (2.2296, -0.8896) (2.5388, -0.8896) (2.9538, -1.286) (2.9538, -1.5557) knots 0 0 0 1 2 2 2
  spline S219 degree 2 poles (2.9538, -1.5557) (2.9538, -1.7487) (2.8646, -1.9417) knots 0 0 0 1 1 1
  spline S220 degree 2 poles (2.8646, -1.9417) (2.7256, -2.2447) (2.4143, -2.585) knots 0 0 0 1 1 1
  spline S221 degree 2 poles (2.4143, -2.585) (1.9474, -3.0934) (1.8312, -3.1993) knots 0 0 0 1 1 1
  line L143 (1.8312, -3.1993) -> (2.4952, -3.1993)
  spline S222 degree 2 poles (2.4952, -3.1993) (2.6986, -3.1993) (2.8605, -3.1702) (2.9912, -3.0768) (3.041, -2.9938) knots 0 0 0 1 2 3 3 3
  line L144 (3.041, -2.9938) -> (3.1095, -2.9938)
  line L145 (4.9916, -0.8896) -> (4.9916, -0.9581)
  spline S223 degree 2 poles (4.9916, -0.9581) (4.7447, -0.983) (4.4293, -1.1303) (4.1242, -1.4333) (3.9229, -1.8068) (3.8545, -2.0642) knots 0 0 0 1 2 3 4 4 4
  spline S224 degree 2 poles (3.8545, -2.0642) (4.1263, -1.8774) (4.3981, -1.8774) knots 0 0 0 1 1 1
  spline S225 degree 2 poles (4.3981, -1.8774) (4.6575, -1.8774) (5.0414, -2.2966) (5.0414, -2.6265) knots 0 0 0 1 2 2 2
  spline S226 degree 2 poles (5.0414, -2.6265) (5.0414, -2.944) (4.8485, -3.2076) knots 0 0 0 1 1 1
  spline S227 degree 2 poles (4.8485, -3.2076) (4.616, -3.5251) (4.2321, -3.5251) knots 0 0 0 1 1 1
  spline S228 degree 2 poles (4.2321, -3.5251) (3.9727, -3.5251) (3.7901, -3.3528) knots 0 0 0 1 1 1
  spline S229 degree 2 poles (3.7901, -3.3528) (3.4332, -3.0187) (3.4332, -2.4833) knots 0 0 0 1 1 1
  spline S230 degree 2 poles (3.4332, -2.4833) (3.4332, -2.143) (3.7071, -1.5288) (4.2155, -1.0535) (4.6824, -0.8896) (4.8837, -0.8896) knots 0 0 0 1 2 3 4 4 4
  line L146 (4.8837, -0.8896) -> (4.9916, -0.8896)
  spline S231 degree 2 poles (3.8233, -2.2011) (3.7901, -2.4522) (3.7901, -2.6078) knots 0 0 0 1 1 1
  spline S232 degree 2 poles (3.7901, -2.6078) (3.7901, -2.7863) (3.9229, -3.2076) (4.0537, -3.3321) knots 0 0 0 1 2 2 2
  spline S233 degree 2 poles (4.0537, -3.3321) (4.1512, -3.4192) (4.2882, -3.4192) knots 0 0 0 1 1 1
  spline S234 degree 2 poles (4.2882, -3.4192) (4.45, -3.4192) (4.7073, -3.1121) (4.7073, -2.8278) knots 0 0 0 1 2 2 2
  spline S235 degree 2 poles (4.7073, -2.8278) (4.7073, -2.5082) (4.4521, -2.0413) (4.2176, -2.0413) knots 0 0 0 1 2 2 2
  spline S236 degree 2 poles (4.2176, -2.0413) (4.1471, -2.0413) (3.9831, -2.1015) (3.8233, -2.2011) knots 0 0 0 1 2 2 2
  line L147 (6.2616, -0.817) -> (5.3423, -3.5334)
  line L148 (5.3423, -3.5334) -> (5.1929, -3.5334)
  line L149 (5.1929, -3.5334) -> (6.1122, -0.817)
  line L150 (6.1122, -0.817) -> (6.2616, -0.817)
  line L151 (8.0152, -2.9938) -> (7.8367, -3.4815)
  line L152 (7.8367, -3.4815) -> (6.3384, -3.4815)
  line L153 (6.3384, -3.4815) -> (6.3384, -3.413)
  spline S237 degree 2 poles (6.3384, -3.413) (7.0004, -2.8091) (7.5399, -2.0455) (7.5399, -1.728) knots 0 0 0 1 2 2 2
  spline S238 degree 2 poles (7.5399, -1.728) (7.5399, -1.4873) (7.2432, -1.176) (7.0378, -1.176) knots 0 0 0 1 2 2 2
  spline S239 degree 2 poles (7.0378, -1.176) (6.8489, -1.176) (6.5522, -1.396) (6.4795, -1.6076) knots 0 0 0 1 2 2 2
  line L154 (6.4795, -1.6076) -> (6.4111, -1.6076)
  spline S240 degree 2 poles (6.4111, -1.6076) (6.4588, -1.2611) (6.8448, -0.8896) (7.1353, -0.8896) knots 0 0 0 1 2 2 2
  spline S241 degree 2 poles (7.1353, -0.8896) (7.4445, -0.8896) (7.8595, -1.286) (7.8595, -1.5557) knots 0 0 0 1 2 2 2
  spline S242 degree 2 poles (7.8595, -1.5557) (7.8595, -1.7487) (7.7703, -1.9417) knots 0 0 0 1 1 1
  spline S243 degree 2 poles (7.7703, -1.9417) (7.6313, -2.2447) (7.32, -2.585) knots 0 0 0 1 1 1
  spline S244 degree 2 poles (7.32, -2.585) (6.8531, -3.0934) (6.7369, -3.1993) knots 0 0 0 1 1 1
  line L155 (6.7369, -3.1993) -> (7.4009, -3.1993)
  spline S245 degree 2 poles (7.4009, -3.1993) (7.6043, -3.1993) (7.7661, -3.1702) (7.8969, -3.0768) (7.9467, -2.9938) knots 0 0 0 1 2 3 3 3
  line L156 (7.9467, -2.9938) -> (8.0152, -2.9938)
  spline S246 degree 2 poles (8.314, -2.226) (8.314, -1.7923) (8.5755, -1.1656) (8.7933, -1.012) knots 0 0 0 1 2 2 2
  spline S247 degree 2 poles (8.7933, -1.012) (8.9614, -0.8896) (9.142, -0.8896) knots 0 0 0 1 1 1
  spline S248 degree 2 poles (9.142, -0.8896) (9.4346, -0.8896) (9.667, -1.1864) knots 0 0 0 1 1 1
  spline S249 degree 2 poles (9.667, -1.1864) (9.9575, -1.5557) (9.9575, -2.1866) knots 0 0 0 1 1 1
  spline S250 degree 2 poles (9.9575, -2.1866) (9.9575, -2.6286) (9.7023, -3.247) (9.308, -3.5251) (9.1233, -3.5251) knots 0 0 0 1 2 3 3 3
  spline S251 degree 2 poles (9.1233, -3.5251) (8.7601, -3.5251) (8.5173, -3.0955) knots 0 0 0 1 1 1
  spline S252 degree 2 poles (8.5173, -3.0955) (8.314, -2.7344) (8.314, -2.226) knots 0 0 0 1 1 1
  spline S253 degree 2 poles (8.6813, -2.2737) (8.6813, -2.7967) (8.8099, -3.1287) knots 0 0 0 1 1 1
  spline S254 degree 2 poles (8.8099, -3.1287) (8.9179, -3.4068) (9.1295, -3.4068) knots 0 0 0 1 1 1
  spline S255 degree 2 poles (9.1295, -3.4068) (9.2312, -3.4068) (9.447, -3.2262) (9.5031, -3.0125) knots 0 0 0 1 2 2 2
  spline S256 degree 2 poles (9.5031, -3.0125) (9.5902, -2.6909) (9.5902, -2.1057) knots 0 0 0 1 1 1
  spline S257 degree 2 poles (9.5902, -2.1057) (9.5902, -1.6699) (9.501, -1.3814) knots 0 0 0 1 1 1
  spline S258 degree 2 poles (9.501, -1.3814) (9.4325, -1.1656) (9.3267, -1.0764) knots 0 0 0 1 1 1
  spline S259 degree 2 poles (9.3267, -1.0764) (9.2499, -1.0141) (9.1399, -1.0141) knots 0 0 0 1 1 1
  spline S260 degree 2 poles (9.1399, -1.0141) (9.0133, -1.0141) (8.9137, -1.1283) knots 0 0 0 1 1 1
  spline S261 degree 2 poles (8.9137, -1.1283) (8.7788, -1.2839) (8.6813, -1.95) (8.6813, -2.2737) knots 0 0 0 1 2 2 2
  line L157 (11.8542, -2.9938) -> (11.6757, -3.4815)
  line L158 (11.6757, -3.4815) -> (10.1775, -3.4815)
  line L159 (10.1775, -3.4815) -> (10.1775, -3.413)
  spline S262 degree 2 poles (10.1775, -3.413) (10.8395, -2.8091) (11.379, -2.0455) (11.379, -1.728) knots 0 0 0 1 2 2 2
  spline S263 degree 2 poles (11.379, -1.728) (11.379, -1.4873) (11.0823, -1.176) (10.8768, -1.176) knots 0 0 0 1 2 2 2
  spline S264 degree 2 poles (10.8768, -1.176) (10.688, -1.176) (10.3912, -1.396) (10.3186, -1.6076) knots 0 0 0 1 2 2 2
  line L160 (10.3186, -1.6076) -> (10.2501, -1.6076)
  spline S265 degree 2 poles (10.2501, -1.6076) (10.2978, -1.2611) (10.6838, -0.8896) (10.9743, -0.8896) knots 0 0 0 1 2 2 2
  spline S266 degree 2 poles (10.9743, -0.8896) (11.2835, -0.8896) (11.6986, -1.286) (11.6986, -1.5557) knots 0 0 0 1 2 2 2
  spline S267 degree 2 poles (11.6986, -1.5557) (11.6986, -1.7487) (11.6093, -1.9417) knots 0 0 0 1 1 1
  spline S268 degree 2 poles (11.6093, -1.9417) (11.4703, -2.2447) (11.159, -2.585) knots 0 0 0 1 1 1
  spline S269 degree 2 poles (11.159, -2.585) (10.6921, -3.0934) (10.5759, -3.1993) knots 0 0 0 1 1 1
  line L161 (10.5759, -3.1993) -> (11.24, -3.1993)
  spline S270 degree 2 poles (11.24, -3.1993) (11.4433, -3.1993) (11.6052, -3.1702) (11.7359, -3.0768) (11.7857, -2.9938) knots 0 0 0 1 2 3 3 3
  line L162 (11.7857, -2.9938) -> (11.8542, -2.9938)
  line L163 (13.7364, -0.8896) -> (13.7364, -0.9581)
  spline S271 degree 2 poles (13.7364, -0.9581) (13.4894, -0.983) (13.174, -1.1303) (12.869, -1.4333) (12.6677, -1.8068) (12.5992, -2.0642) knots 0 0 0 1 2 3 4 4 4
  spline S272 degree 2 poles (12.5992, -2.0642) (12.871, -1.8774) (13.1429, -1.8774) knots 0 0 0 1 1 1
  spline S273 degree 2 poles (13.1429, -1.8774) (13.4023, -1.8774) (13.7862, -2.2966) (13.7862, -2.6265) knots 0 0 0 1 2 2 2
  spline S274 degree 2 poles (13.7862, -2.6265) (13.7862, -2.944) (13.5932, -3.2076) knots 0 0 0 1 1 1
  spline S275 degree 2 poles (13.5932, -3.2076) (13.3608, -3.5251) (12.9769, -3.5251) knots 0 0 0 1 1 1
  spline S276 degree 2 poles (12.9769, -3.5251) (12.7175, -3.5251) (12.5349, -3.3528) knots 0 0 0 1 1 1
  spline S277 degree 2 poles (12.5349, -3.3528) (12.1779, -3.0187) (12.1779, -2.4833) knots 0 0 0 1 1 1
  spline S278 degree 2 poles (12.1779, -2.4833) (12.1779, -2.143) (12.4519, -1.5288) (12.9603, -1.0535) (13.4272, -0.8896) (13.6285, -0.8896) knots 0 0 0 1 2 3 4 4 4
  line L164 (13.6285, -0.8896) -> (13.7364, -0.8896)
  spline S279 degree 2 poles (12.5681, -2.2011) (12.5349, -2.4522) (12.5349, -2.6078) knots 0 0 0 1 1 1
  spline S280 degree 2 poles (12.5349, -2.6078) (12.5349, -2.7863) (12.6677, -3.2076) (12.7984, -3.3321) knots 0 0 0 1 2 2 2
  spline S281 degree 2 poles (12.7984, -3.3321) (12.8959, -3.4192) (13.0329, -3.4192) knots 0 0 0 1 1 1
  spline S282 degree 2 poles (13.0329, -3.4192) (13.1948, -3.4192) (13.4521, -3.1121) (13.4521, -2.8278) knots 0 0 0 1 2 2 2
  spline S283 degree 2 poles (13.4521, -2.8278) (13.4521, -2.5082) (13.1968, -2.0413) (12.9623, -2.0413) knots 0 0 0 1 2 2 2
  spline S284 degree 2 poles (12.9623, -2.0413) (12.8918, -2.0413) (12.7279, -2.1015) (12.5681, -2.2011) knots 0 0 0 1 2 2 2
  point P0 (0, 14.35)
  point P1 (-13.5728, 0.5359)
  constraints: 1 other
emboss "Emboss5" sketch "Sketch19" operation cut depth 5 direction (0, 0, -1) wrap yes faces at (12.1913, -14.3543, 27.2195)
body "Solid1"
